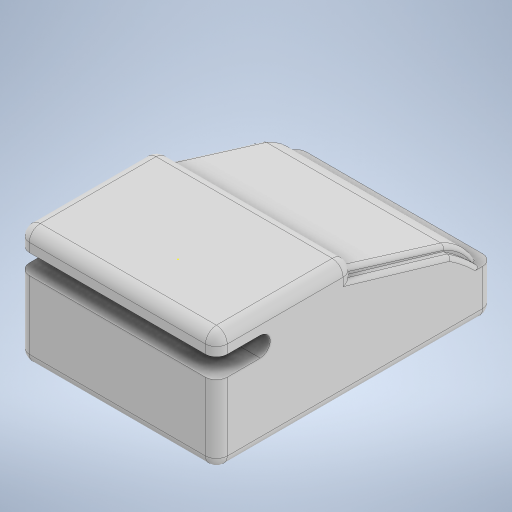
# Autodesk Inventor part: base
Saved by Autodesk Inventor 2024 (Build 280153000, 153)
## iProperties
Created: 2023-07-11
Part Number: base
Material: Generic
Document SubType Name: Modeling
Designer: KSABD
Density: 1 g/cm^3
Appearance: Default
Author: KSABD
Autodesk Inventor part; units mm, degrees
ref_plane "YZ Plane" through (0, 0, 0) normal (1, 0, 0) x (0, 1, 0)
ref_plane "XZ Plane" through (0, 0, 0) normal (0, 1, 0) x (-1, 0, 0)
ref_plane "XY Plane" through (0, 0, 0) normal (0, 0, 1) x (1, 0, 0)
sketch "Sketch1" plane through (0, 0, 0) normal (0, 0, 1) x (1, 0, 0)
  line L0 (-857.5583, 393.3301) -> (412.4417, 393.3301)
  line L1 (412.4417, 393.3301) -> (412.4417, -368.6699)
  line L2 (412.4417, -368.6699) -> (-857.5583, -368.6699)
  line L3 (-857.5583, -368.6699) -> (-857.5583, 393.3301)
  point P0 (0, 0)
  dimension "d1" = 762
  dimension "d2" = 1270
  constraints: 8 end point, 2 parallel, 1 horizontal, 1 perpendicular
  measures "d1" distance of L0.end L1.end
  measures "d2" distance of L1.end L2.end
extrude "Extrusion1" add sketch "Sketch1" against normal blind 1778
sketch "Sketch2" plane through (-857.5583, -368.6699, 0) normal (-1, 0, 0) x (0, 0, 1)
  line L0 (-1778, 0) -> (-1778, 762) projected
  line L1 (-1778, 304.8) -> (-889, 304.8)
  line L2 (-889, 304.8) -> (-889, 762)
  line L3 (0, 762) -> (-1778, 762) projected
  line L4 (0, 762) -> (0, 0) projected
  line L5 (0, 0) -> (-1778, 0) projected
  line L6 (-1778, 304.8) -> (-1778, 762)
  line L7 (-889, 762) -> (-1778, 762)
  point P0 (0, 368.6699)
  dimension "d5" = 889
  dimension "d6" = 304.8
  constraints: 8 end point, 2 perpendicular, 1 collinear, 1 midpoint, 1 point on line, 1 vertical
  measures "d5" distance between parallel lines of L4 L2
  measures "d6" distance between parallel lines of L5 L1
extrude "Extrusion2" cut sketch "Sketch2" against normal blind 1778 contours L0 L3 L2 L1
fillet "Fillet1" radius 70 9 edges at (-857.5583, 12.3301, 0) (-857.5583, -216.2699, -1778) (-857.5583, 393.3301, -444.5) (412.4417, 12.3301, 0) (-857.5583, -368.6699, -889) (-222.5583, -368.6699, 0) (-222.5583, 393.3301, 0) (412.4417, 393.3301, -444.5) (412.4417, -368.6699, -889)
fillet "Fillet2" radius 70 4 edges at (391.9392, -348.1674, -1778) (-222.5583, -368.6699, -1778) (-837.0557, -348.1674, -1757.4975) (412.4417, -181.2699, -1778)
sketch "Sketch3" plane through (-857.5583, -298.6699, -70) normal (-1, 0, 0) x (0, 0, 1)
  line L0 (-819, 234.8) -> (-819, 622) projected
  line L1 (-819, 234.8) -> (-1638, 234.8) projected
  arc A0 (-818.9715, 575.3412) -> (-819, 575.3417) centre (-835.9403, -520.1831) ccw
  arc A1 (-1435.8249, 392.2509) -> (-1626.0778, 233.5278) centre (-835.9403, -520.1831) ccw
  arc A2 (-819.1112, 571.6585) -> (-818.9715, 575.3412) centre (-819, 573.4983) ccw
  arc A3 (-1628.7481, 236.0691) -> (-1626.0778, 233.5278) centre (-1627.4115, 234.8) ccw
  arc A4 (-819, 573.4983) -> (-820.843, 573.5253) centre (-835.9403, -520.1831) ccw construction
  arc A5 (-1435.8249, 394.4559) -> (-1627.4115, 234.8) centre (-835.9403, -520.1831) ccw construction
  line L2 (-781.363, 570.4216) -> (-819, 575.3417)
  line L3 (-1435.8249, 392.2509) -> (-819, 573.4983)
  point P0 (70, 298.6699)
  point P1 (-1624.8623, 234.8)
  constraints: 14 point on circle, 6 centre point, 4 end point, 4 tangent, 3 point on line
extrude "Extrusion3" add sketch "Sketch3" against normal blind 1270 contours L0 L1 A1 L3
fillet "Fillet3" radius 25.4 4 edges at (-857.5583, 20.1963, -1604.7919) (-857.5583, 184.2047, -1197.4124) (412.4417, 184.2047, -1197.4124) (412.4417, 20.1963, -1604.7919)
fillet "Fillet4" radius 76.2 7 edges at (-837.0557, 372.8276, -889) (-222.5583, 393.3301, -889) (391.9392, 372.8276, -889) (412.4417, 261.5915, -889) (412.4417, 299.0793, -889) (-857.5583, 261.5915, -889) (-857.5583, 299.0793, -889)
ref_plane "Work Plane1" through (-806.7583, 254.4933, -868.1085) normal (-1, 0, 0) x (0, 0, 1)
sketch "Sketch6" plane through (-806.7583, 254.4933, -868.1085) normal (-1, 0, 0) x (0, 0, 1)
  line L0 (-20.8915, 62.6368) -> (-20.8915, 20.3351) projected
  line L1 (-909.8915, -318.3632) -> (-839.8915, -318.3632) projected
  arc A0 (-646.5442, -129.9407) -> (-851.94, -318.3632) centre (-489.7051, -507.0685) ccw
  line L2 (-646.5442, -129.9407) -> (-20.8915, 62.6368)
  arc A1 (-637.7163, -160.9123) -> (-826.7537, -318.3632) centre (-37.8318, -1073.3463) ccw projected
  line L3 (-851.94, -318.3632) -> (-826.7537, -318.3632)
  line L4 (-851.94, -318.3632) -> (-826.7537, -318.3632)
  line L5 (-637.7163, -160.9123) -> (-20.8915, 20.3351)
  ellipse E0 centre (55.3085, 62.6368) end of major axis (131.5085, 62.6368) minor radius 6.2 (55.3085, 68.8368) -> (-20.8915, 62.6368) ccw projected
  line L6 (-20.8915, 20.3351) -> (-1.4876, 26.0367) projected
  line L7 (-20.8915, 62.6368) -> (-20.8915, 20.3351)
  line L8 (-20.8915, 20.3351) -> (-637.7163, -160.9123)
  arc A2 (-637.7163, -160.9123) -> (-826.7537, -318.3632) centre (-37.8318, -1073.3463) ccw
  point P0 (868.1085, -254.4933)
  constraints: 12 end point, 4 point on circle, 2 centre point, 2 collinear, 1 concentric, 1 horizontal, 1 point on line, 1 vertical, 1 other
extrude "Extrusion4" add sketch "Sketch6" against normal blind 1168.4
sketch "Sketch7" plane through (-806.7583, 124.5526, -1514.6527) normal (0, 0.9557494, -0.2941821) x (1, 0, 0)
  point P0 (806.7583, -1410.9872)
fillet "Fillet8" radius 25.4 4 edges at (361.6417, 220.8413, -1201.8264) (361.6417, 48.4042, -1633.9209) (-806.7583, 220.8413, -1201.8264) (-806.7583, 48.4042, -1633.9209)
sketch "Sketch8" plane through (-857.5583, -298.6699, -70) normal (-1, 0, 0) x (0, 0, 1)
  line L0 (70, 0) -> (70, 622) projected
  line L1 (70, 438) -> (-223.907, 438)
  line L2 (70, 565) -> (47.9145, 565)
  line L3 (47.9145, 565) -> (-211.4485, 565)
  line L4 (0, 692) -> (-742.8, 692) projected
  arc A0 (-211.4485, 565) -> (-211.4485, 438) centre (-211.4485, 501.5) ccw
  point P0 (70, 298.6699)
  dimension "d21" = 127
  dimension "d22" = 127
  constraints: 6 end point, 4 point on line, 2 point on circle, 2 tangent, 1 centre point, 1 horizontal, 1 perpendicular
  measures "d21" distance between parallel lines of L4 L3
  measures "d22" distance between parallel lines of L3 L1
extrude "Extrusion5" cut sketch "Sketch8" against normal blind 1270
body "Solid1"
